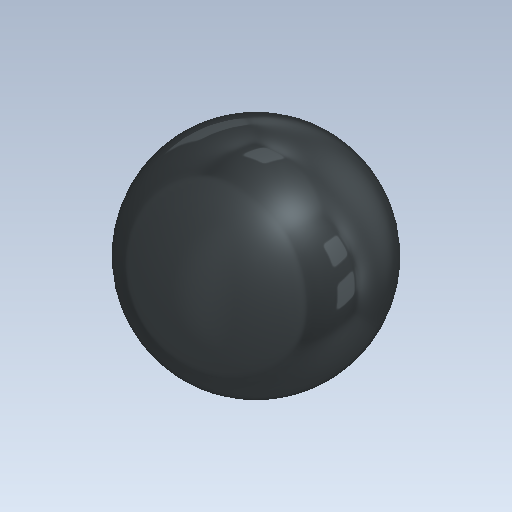
# Autodesk Inventor part: 20-47-31-14-ybrg1-47-7.938-33.5
Saved by Autodesk Inventor 2020 (Build 240168000, 168)
## iProperties
Part Number: 20-47-31-14-ybrg1-47-7.938-33.5
Material: Iron, Cast
Catalog Web Link: www.cadenas.de
Description: Ball for Y units-Y-bearings
Vendor: SKF
Document SubType Name: Modeling
Designer: partserver
Manufacturer: SKF
Mass: 1.87257 g
Surface Area: 1.97958 cm^2
Volume: 0.261898 cm^3
Density: 7.15 g/cm^3
Appearance: Iron Gray
Category: PARTsolutions
Company: SKF
PSOL_IDENT_0: {$CADENAS_DATA\23d-libs\skf\bearings_units_and_housings\bearing_units\ball_bearing_units\y-unit_acce
PSOL_IDENT_1: ssories\ball.prj},214 {VTYP=3D},{NB=20-47-31-14-ybrg1-47-7.938-33.5},{LINA=20-47-31-14-ybrg1-47-7.93
PSOL_IDENT_2: 8-33.5},{NN=Ball for Y units},{DATE=20.08.2020 13:45:09},{GEOMDATE=29.07.2020 16:06:32},{VERSION=},{
PSOL_IDENT_3: LINEID=1140},{WBVAR=},{WBNUMERIC=}  {NB=20-47-31-14-ybrg1-47-7.938-33.5},{LINA=20-47-31-14-ybrg1-47-
PSOL_IDENT_4: 7.938-33.5},{KT=DUMMY},{DD=20.0000},{D=47},{B=31.000},{C=14.000},{PITCH=33.500},{DW=7.938},{FO=IEC_B
PSOL_IDENT_5: BY_006},{DESIGN=ybrg1},{X=0},{PN=47}
NB: 20-47-31-14-ybrg1-47-7.938-33.5
NN: Ball for Y units
NT: Y-bearings
NBSYN: $DD.-$D.-$B.-$C.-$DESIGN.-$PN.-$DW.-$PITCH.
LINA: 20-47-31-14-ybrg1-47-7.938-33.5
CATALOG: SKF
DD: 20
D: 47
B: 31
C: 14
PITCH: 33.5
DW: 7.938
FO: IEC_BBY_006
DESIGN: ybrg1
SUPPLIER: SKF
ARTICLENO: 20-47-31-14-ybrg1-47-7.938-33.5
BOMINFO: 20-47-31-14-ybrg1-47-7.938-33.5
CREATOR: CADENAS GmbH
Title: 20-47-31-14-ybrg1-47-7.938-33.5
Author: Cadenas PARTsolutions
Comments: Y-bearings
Autodesk Inventor part; units mm, degrees
sketch "Sketch_1" plane through (0, 0, 0) normal (0, 0, 1) x (1, 0, 0)
  line L0 (3.969, 16.75) -> (-3.969, 16.75)
  arc A0 (3.969, 16.75) -> (-3.969, 16.75) centre (0, 16.75) ccw
  line L1 (3.969, 16.75) -> (-3.969, 16.75)
  constraints: 4 end point, 2 point on circle, 1 centre point
revolve "Revolution1" add sketch "Sketch_1" angle 360 about axis through (3.969, 16.75, 0) along (1, 0, 0)
ref_plane "ball_XY" through (0, 16.75, 0) normal (1, 0, 0) x (0, 0, -1)
ref_plane "ball_YZ" through (0, 16.75, 0) normal (0, 0, -1) x (0, 1, 0)
ref_plane "ball_ZX" through (0, 16.75, 0) normal (0, 1, 0) x (1, 0, 0)
body "Solid1"
